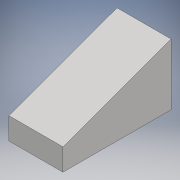
# Autodesk Inventor part: Halter
Saved by Autodesk Inventor 2017.3 (Build 213257000, 257)
## iProperties
Created: 2019-08-08
Part Number: Halter
Material: Generic
Document SubType Name: Modeling
Designer: Ole Simmering
Density: 1 g/cm^3
Appearance: Default
Author: Ole Simmering
Autodesk Inventor part; units mm, degrees
ref_plane "YZ Plane" through (0, 0, 0) normal (1, 0, 0) x (0, 1, 0)
ref_plane "XZ Plane" through (0, 0, 0) normal (0, 1, 0) x (-1, 0, 0)
ref_plane "XY Plane" through (0, 0, 0) normal (0, 0, 1) x (1, 0, 0)
sketch "Sketch1" plane through (0, 0, 0) normal (0, 0, 1) x (1, 0, 0)
  line L0 (0, 0) -> (15, 0)
  line L1 (15, 0) -> (15, 30)
  line L2 (15, 30) -> (0, 30)
  line L3 (0, 30) -> (0, 0)
  dimension "d0" = 30
  dimension "d1" = 15
  constraints: 8 end point, 2 parallel, 1 horizontal, 1 perpendicular
  measures "d0" distance of L1.end L0.end
  measures "d1" distance of L1.end L2.end
extrude "Extrusion1" add sketch "Sketch1" along normal blind 17
sketch "Sketch2" plane through (15, 0, 0) normal (1, 0, 0) x (0, 0, -1)
  line L0 (-17, 0) -> (-17, 30) projected
  line L1 (-17, 30) -> (-6.0809, 0)
  line L2 (-17, 30) -> (14.9253, 30) construction
  line L3 (-6.0809, 0) -> (-17, 0)
  line L4 (-6.0809, 0) -> (-17, 0)
  line L5 (-17, 30) -> (-17, 0)
  dimension "d4" = 70
  constraints: 10 end point, 2 collinear, 1 equal length, 1 horizontal
  measures "d4" angle of L1 L2
extrude "Extrusion2" cut sketch "Sketch2" against normal through all
sketch "Sketch3" plane through (0, 30, 0) normal (0, 1, 0) x (1, 0, 0)
  circle A0 centre (7.5, -7.5) radius 3.9624
  line L0 (15, -17) -> (0, -17) construction
  line L1 (7.5, -17) -> (7.5, 2) construction
  line L2 (0, 0) -> (0, -17) construction
  line L3 (0, -8.5) -> (15, -8.5) construction
  dimension "d7" = 7.9248
  constraints: 4 end point, 3 midpoint, 2 perpendicular, 1 centre point, 1 coincident
  measures "d7" diameter of A0
hole "Hole1" at (7.5, 30, 7.5) direction (0, -1, 0) diameter 7.9248 depth 12.7 tip angle 118
body "Solid1"
